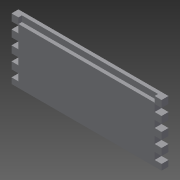
# Autodesk Inventor part: deep_end
Saved by Autodesk Inventor 2014 SP1 (Build 180222100, 222)
## iProperties
Created: 2014-02-23
Part Number: deep_end
Material: Wood (Birch)
Document SubType Name: Modeling
Designer: Chris
Density: 0.55 g/cm^3
Appearance: Birch - Natural Polished
Mass: 666.144 g
Surface Area: 1613.5 cm^2
Volume: 1211.17 cm^3
Author: Chris
Autodesk Inventor part; units mm, degrees
ref_plane "YZ Plane" through (0, 0, 0) normal (1, 0, 0) x (0, 1, 0)
ref_plane "XZ Plane" through (0, 0, 0) normal (0, 1, 0) x (-1, 0, 0)
ref_plane "XY Plane" through (0, 0, 0) normal (0, 0, 1) x (1, 0, 0)
sketch "Sketch1" plane through (0, 0, 0) normal (0, 0, 1) x (1, 0, 0)
  line L0 (0, 244.475) -> (19.05, 244.475)
  line L1 (19.05, 244.475) -> (19.05, 225.425)
  line L2 (19.05, 225.425) -> (0, 225.425)
  line L3 (0, 225.425) -> (0, 244.475)
  line L4 (19.05, 168.275) -> (0, 168.275)
  line L5 (0, 168.275) -> (0, 149.225)
  line L6 (0, 149.225) -> (19.05, 149.225)
  line L7 (19.05, 149.225) -> (19.05, 168.275)
  line L8 (0, 130.175) -> (19.05, 130.175)
  line L9 (19.05, 130.175) -> (19.05, 111.125)
  line L10 (19.05, 111.125) -> (0, 111.125)
  line L11 (0, 111.125) -> (0, 130.175)
  line L12 (0, 206.375) -> (19.05, 206.375)
  line L13 (19.05, 206.375) -> (19.05, 187.325)
  line L14 (19.05, 187.325) -> (0, 187.325)
  line L15 (0, 187.325) -> (0, 206.375)
  line L16 (0, 92.075) -> (19.05, 92.075)
  line L17 (19.05, 92.075) -> (19.05, 73.025)
  line L18 (19.05, 73.025) -> (0, 73.025)
  line L19 (0, 73.025) -> (0, 92.075)
  line L20 (0, 53.975) -> (19.05, 53.975)
  line L21 (19.05, 53.975) -> (19.05, 34.925)
  line L22 (19.05, 34.925) -> (0, 34.925)
  line L23 (0, 34.925) -> (0, 53.975)
  line L24 (0, 15.875) -> (19.05, 15.875)
  line L25 (19.05, 15.875) -> (19.05, -3.175)
  line L26 (19.05, -3.175) -> (0, -3.175)
  line L27 (0, -3.175) -> (0, 15.875)
  line L28 (0, 244.475) -> (206.375, 244.475)
  line L29 (206.375, 244.475) -> (206.375, 76.2)
  line L30 (206.375, 76.2) -> (0, 76.2)
  line L31 (19.05, 244.475) -> (19.05, 76.2)
  line L32 (206.375, 244.475) -> (19.05, 244.475)
  line L33 (19.05, 244.475) -> (19.05, 76.2)
  line L34 (19.05, 76.2) -> (206.375, 76.2)
  line L35 (206.375, 76.2) -> (206.375, 244.475)
  line L36 (0, 92.075) -> (19.05, 92.075)
  line L37 (19.05, 92.075) -> (19.05, 76.2)
  line L38 (19.05, 76.2) -> (0, 76.2)
  line L39 (0, 76.2) -> (0, 92.075)
  dimension "d0" = 19.05
  dimension "d1" = 19.05
  dimension "d3" = 19.05
  dimension "d4" = 19.05
  dimension "d5" = 19.05
  dimension "d6" = 19.05
  dimension "d7" = 19.05
  dimension "d8" = 19.05
  dimension "d9" = 19.05
  dimension "d10" = 19.05
  dimension "d11" = 19.05
  dimension "d12" = 19.05
  dimension "d13" = 19.05
  dimension "d14" = 19.05
  dimension "d15" = 19.05
  dimension "d16" = 19.05
  dimension "d17" = 19.05
  dimension "d18" = 19.05
  dimension "d19" = 19.05
  dimension "d21" = 206.375
  dimension "d22" = 168.275
  dimension "d23" = 206.375
  constraints: 80 end point, 18 parallel, 12 perpendicular, 9 horizontal, 3 point on line
  measures "d0" distance of L0.end L1.end
  measures "d1" distance of L1.end L2.end
  measures "d3" distance between parallel lines of L12 L2
  measures "d4" distance between parallel lines of L14 L12
  measures "d5" distance between parallel lines of L4 L14
  measures "d6" distance between parallel lines of L6 L4
  measures "d7" distance between parallel lines of L8 L6
  measures "d8" distance of L8.end L9.end
  measures "d9" distance of L12.start L12.end
  measures "d10" distance of L4.start L4.end
  measures "d11" distance of L8.start L8.end
  measures "d12" distance between parallel lines of L10 L16
  measures "d13" distance of L16.end L17.end
  measures "d14" distance between parallel lines of L18 L20
  measures "d15" distance of L20.end L21.end
  measures "d16" distance of L24.start L24.end
  measures "d17" distance between parallel lines of L24 L22
  measures "d18" distance of L25.end L26.end
  measures "d19" distance between parallel lines of L24 L26
  measures "d21" distance of L0.start L28.end
  measures "d22" distance of L28.end L29.end
  measures "d23" distance of L29.end L30.end
extrude "Extrusion3" add sketch "Sketch1" along normal blind 19.05 contours L0 L1 L2 L3 | L28 L29 L30 L17 L31 L9 L7 L13 L1 | L13 L14 L15 L12 | L30 L19 L16 L17 | L7 L6 L5 L4 | L10 L11 L8 L9
mirror "Mirror2" about plane through (206.375, 76.2, 0) normal (1, 0, 0) of "Extrusion3"
sketch "Sketch3" plane through (0, 0, 19.05) normal (0, 0, 1) x (1, 0, 0)
  line L0 (0, 244.475) -> (412.75, 244.475) projected
  line L1 (19.05, 244.475) -> (393.7, 244.475)
  line L2 (393.7, 244.475) -> (393.7, 228.6)
  line L3 (393.7, 228.6) -> (19.05, 228.6)
  line L4 (19.05, 228.6) -> (19.05, 244.475)
  point P0 (0, 0)
  dimension "d33" = 15.875
  constraints: 8 end point, 2 parallel, 1 horizontal, 1 perpendicular, 1 point on line
  measures "d33" distance of L3.end L1.start
extrude "Extrusion4" cut sketch "Sketch3" against normal blind 9.525
body "Solid2"
